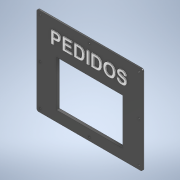
# Autodesk Inventor part: Front_Plate
Saved by Autodesk Inventor 2020 (Build 240168000, 168)
## iProperties
Created: 2020-06-21
Part Number: Front_Plate
Material: Generic
Document SubType Name: Modeling
Designer: Erick Miranda
Density: 1 g/cm^3
Appearance: Anodized - Black
Author: Erick Miranda
Autodesk Inventor part; units mm, degrees
ref_plane "YZ Plane" through (0, 0, 0) normal (1, 0, 0) x (0, 1, 0)
ref_plane "XZ Plane" through (0, 0, 0) normal (0, 1, 0) x (-1, 0, 0)
ref_plane "XY Plane" through (0, 0, 0) normal (0, 0, 1) x (1, 0, 0)
sketch "Sketch1" plane through (0, 0, 0) normal (0, 0, 1) x (1, 0, 0)
  line L0 (0, 0) -> (300, 0)
  line L1 (300, 0) -> (300, 250)
  line L2 (300, 250) -> (0, 250)
  line L3 (0, 250) -> (0, 0)
  dimension "d0" = 300
  dimension "d1" = 250
  constraints: 8 end point, 2 parallel, 1 horizontal, 1 perpendicular
  measures "d0" distance of L0.start L0.end
  measures "d1" distance of L0.end L1.end
extrude "Extrusion1" add sketch "Sketch1" along normal blind 4
fillet "Fillet1" radius 5 4 edges at (300, 250, 2) (0, 250, 2) (300, 0, 2) (0, 0, 2)
sketch "Sketch5" plane through (0, 0, 4) normal (0, 0, 1) x (1, 0, 0)
  line L0 (5, 0) -> (295, 0) projected
  line L1 (150, 0) -> (150, 33.5)
  line L2 (150, 33.5) -> (240.075, 33.5)
  line L3 (150, 33.5) -> (59.925, 33.5)
  line L4 (240.075, 33.5) -> (240.075, 155.5)
  line L5 (240.075, 155.5) -> (59.925, 155.5)
  line L6 (59.925, 155.5) -> (59.925, 33.5)
  point P0 (0, 0)
  dimension "d54" = 33.5
  dimension "d55" = 90.075
  dimension "d56" = 90.075
  dimension "d57" = 122
  dimension "d58" = 180.15
  constraints: 12 end point, 2 horizontal, 2 vertical, 1 midpoint, 1 perpendicular
  measures "d54" distance of L1.start L1.end
  measures "d55" distance of L1.end L2.end
  measures "d56" distance of L1.end L3.end
  measures "d57" distance of L2.end L4.end
  measures "d58" distance of L4.end L5.end
extrude "Extrusion5" cut sketch "Sketch5" against normal blind 81.3
chamfer "Chamfer2" distance 4 angle 45 4 edges at (240.075, 94.5, 4) (150, 33.5, 4) (150, 155.5, 4) (59.925, 94.5, 4)
sketch "Sketch7" plane through (0, 0, 4) normal (0, 0, 1) x (1, 0, 0)
  line L0 (38.9812, 222.1743) -> (264.0529, 222.1743) construction
  line L1 (264.0529, 222.1743) -> (264.0529, 185.0338) construction
  line L2 (264.0529, 185.0338) -> (38.9812, 185.0338) construction
  line L3 (38.9812, 185.0338) -> (38.9812, 222.1743) construction
  line L4 (42.5559, 186.5874) -> (42.5559, 221.5874)
  line L5 (42.5559, 221.5874) -> (53.8935, 221.5874)
  spline S0 degree 2 poles (53.8935, 221.5874) (60.3493, 221.5874) (62.2967, 221.0539) knots 0 0 0 1 1 1
  spline S1 degree 2 poles (62.2967, 221.0539) (65.3112, 220.2803) (69.3661, 214.9982) (69.3661, 210.81) knots 0 0 0 1 2 2 2
  spline S2 degree 2 poles (69.3661, 210.81) (69.3661, 207.6088) (67.0185, 203.2071) (63.4172, 200.6995) (61.5498, 200.2993) knots 0 0 0 1 2 3 3 3
  spline S3 degree 2 poles (61.5498, 200.2993) (59.0422, 199.7924) (54.2403, 199.7924) knots 0 0 0 1 1 1
  line L6 (54.2403, 199.7924) -> (49.6253, 199.7924)
  line L7 (49.6253, 199.7924) -> (49.6253, 186.5874)
  line L8 (49.6253, 186.5874) -> (42.5559, 186.5874)
  line L9 (49.6253, 215.6652) -> (49.6253, 205.7147)
  line L10 (49.6253, 205.7147) -> (53.4934, 205.7147)
  spline S4 degree 2 poles (53.4934, 205.7147) (57.6817, 205.7147) (60.4827, 206.8085) (62.0833, 209.156) (62.0833, 210.7033) knots 0 0 0 1 2 3 3 3
  spline S5 degree 2 poles (62.0833, 210.7033) (62.0833, 212.624) (59.8425, 215.1049) (58.1085, 215.4251) knots 0 0 0 1 2 2 2
  spline S6 degree 2 poles (58.1085, 215.4251) (56.8547, 215.6652) (53.0399, 215.6652) knots 0 0 0 1 1 1
  line L11 (53.0399, 215.6652) -> (49.6253, 215.6652)
  line L12 (75.1817, 186.5874) -> (75.1817, 221.5874)
  line L13 (75.1817, 221.5874) -> (101.1382, 221.5874)
  line L14 (101.1382, 221.5874) -> (101.1382, 215.6652)
  line L15 (101.1382, 215.6652) -> (82.251, 215.6652)
  line L16 (82.251, 215.6652) -> (82.251, 207.9022)
  line L17 (82.251, 207.9022) -> (99.831, 207.9022)
  line L18 (99.831, 207.9022) -> (99.831, 201.9799)
  line L19 (99.831, 201.9799) -> (82.251, 201.9799)
  line L20 (82.251, 201.9799) -> (82.251, 192.5097)
  line L21 (82.251, 192.5097) -> (101.8051, 192.5097)
  line L22 (101.8051, 192.5097) -> (101.8051, 186.5874)
  line L23 (101.8051, 186.5874) -> (75.1817, 186.5874)
  line L24 (107.7541, 221.5874) -> (120.6923, 221.5874)
  spline S7 degree 2 poles (120.6923, 221.5874) (125.0673, 221.5874) (127.3615, 220.9205) knots 0 0 0 1 1 1
  spline S8 degree 2 poles (127.3615, 220.9205) (130.4294, 220.0135) (134.831, 215.3717) (137.1253, 208.6758) (137.1253, 203.7406) knots 0 0 0 1 2 3 3 3
  spline S9 degree 2 poles (137.1253, 203.7406) (137.1253, 199.419) (136.0582, 196.2978) knots 0 0 0 1 1 1
  spline S10 degree 2 poles (136.0582, 196.2978) (134.7243, 192.483) (132.2967, 190.1088) knots 0 0 0 1 1 1
  spline S11 degree 2 poles (132.2967, 190.1088) (130.456, 188.3214) (127.3349, 187.3344) knots 0 0 0 1 1 1
  spline S12 degree 2 poles (127.3349, 187.3344) (124.9873, 186.5874) (121.0658, 186.5874) knots 0 0 0 1 1 1
  line L25 (121.0658, 186.5874) -> (107.7541, 186.5874)
  line L26 (107.7541, 186.5874) -> (107.7541, 221.5874)
  line L27 (114.8234, 215.6652) -> (114.8234, 192.5097)
  line L28 (114.8234, 192.5097) -> (120.1054, 192.5097)
  spline S13 degree 2 poles (120.1054, 192.5097) (123.0932, 192.5097) (124.4004, 192.8565) knots 0 0 0 1 1 1
  spline S14 degree 2 poles (124.4004, 192.8565) (126.1344, 193.2833) (128.4019, 195.3107) (129.8425, 200.0325) (129.8425, 204.0874) knots 0 0 0 1 2 3 3 3
  spline S15 degree 2 poles (129.8425, 204.0874) (129.8425, 208.1423) (128.4019, 212.4639) (125.8143, 214.8915) (123.8402, 215.3184) knots 0 0 0 1 2 3 3 3
  spline S16 degree 2 poles (123.8402, 215.3184) (122.3463, 215.6652) (117.998, 215.6652) knots 0 0 0 1 1 1
  line L29 (117.998, 215.6652) -> (114.8234, 215.6652)
  line L30 (142.8875, 186.5874) -> (142.8875, 221.5874)
  line L31 (142.8875, 221.5874) -> (149.9568, 221.5874)
  line L32 (149.9568, 221.5874) -> (149.9568, 186.5874)
  line L33 (149.9568, 186.5874) -> (142.8875, 186.5874)
  line L34 (156.6527, 221.5874) -> (169.591, 221.5874)
  spline S17 degree 2 poles (169.591, 221.5874) (173.966, 221.5874) (176.2602, 220.9205) knots 0 0 0 1 1 1
  spline S18 degree 2 poles (176.2602, 220.9205) (179.328, 220.0135) (183.7297, 215.3717) (186.0239, 208.6758) (186.0239, 203.7406) knots 0 0 0 1 2 3 3 3
  spline S19 degree 2 poles (186.0239, 203.7406) (186.0239, 199.419) (184.9568, 196.2978) knots 0 0 0 1 1 1
  spline S20 degree 2 poles (184.9568, 196.2978) (183.623, 192.483) (181.1954, 190.1088) knots 0 0 0 1 1 1
  spline S21 degree 2 poles (181.1954, 190.1088) (179.3547, 188.3214) (176.2335, 187.3344) knots 0 0 0 1 1 1
  spline S22 degree 2 poles (176.2335, 187.3344) (173.8859, 186.5874) (169.9644, 186.5874) knots 0 0 0 1 1 1
  line L35 (169.9644, 186.5874) -> (156.6527, 186.5874)
  line L36 (156.6527, 186.5874) -> (156.6527, 221.5874)
  line L37 (163.7221, 215.6652) -> (163.7221, 192.5097)
  line L38 (163.7221, 192.5097) -> (169.0041, 192.5097)
  spline S23 degree 2 poles (169.0041, 192.5097) (171.9919, 192.5097) (173.299, 192.8565) knots 0 0 0 1 1 1
  spline S24 degree 2 poles (173.299, 192.8565) (175.033, 193.2833) (177.3006, 195.3107) (178.7411, 200.0325) (178.7411, 204.0874) knots 0 0 0 1 2 3 3 3
  spline S25 degree 2 poles (178.7411, 204.0874) (178.7411, 208.1423) (177.3006, 212.4639) (174.7129, 214.8915) (172.7388, 215.3184) knots 0 0 0 1 2 3 3 3
  spline S26 degree 2 poles (172.7388, 215.3184) (171.2449, 215.6652) (166.8966, 215.6652) knots 0 0 0 1 1 1
  line L39 (166.8966, 215.6652) -> (163.7221, 215.6652)
  spline S27 degree 2 poles (190.5856, 203.874) (190.5856, 209.2094) (192.1862, 212.8374) knots 0 0 0 1 1 1
  spline S28 degree 2 poles (192.1862, 212.8374) (193.3867, 215.5051) (197.5216, 219.7734) (199.9759, 220.7871) knots 0 0 0 1 2 2 2
  spline S29 degree 2 poles (199.9759, 220.7871) (203.2304, 222.1743) (207.5254, 222.1743) knots 0 0 0 1 1 1
  spline S30 degree 2 poles (207.5254, 222.1743) (215.2617, 222.1743) (224.5452, 212.5707) (224.5452, 204.0341) knots 0 0 0 1 2 2 2
  spline S31 degree 2 poles (224.5452, 204.0341) (224.5452, 195.5775) (215.315, 186.0005) (207.6054, 186.0005) knots 0 0 0 1 2 2 2
  spline S32 degree 2 poles (207.6054, 186.0005) (199.8158, 186.0005) (190.5856, 195.5242) (190.5856, 203.874) knots 0 0 0 1 2 2 2
  spline S33 degree 2 poles (197.8684, 204.1141) (197.8684, 198.1652) (203.3638, 192.0295) (207.6054, 192.0295) knots 0 0 0 1 2 2 2
  spline S34 degree 2 poles (207.6054, 192.0295) (211.8471, 192.0295) (217.2625, 198.1118) (217.2625, 204.1941) knots 0 0 0 1 2 2 2
  spline S35 degree 2 poles (217.2625, 204.1941) (217.2625, 210.2231) (211.9804, 216.1453) (207.6054, 216.1453) knots 0 0 0 1 2 2 2
  spline S36 degree 2 poles (207.6054, 216.1453) (203.2304, 216.1453) (197.8684, 210.1431) (197.8684, 204.1141) knots 0 0 0 1 2 2 2
  line L40 (228.2533, 198.0051) -> (235.1359, 198.672)
  spline S37 degree 2 poles (235.1359, 198.672) (235.7495, 195.204) (239.5643, 191.9495) (242.7655, 191.9495) knots 0 0 0 1 2 2 2
  spline S38 degree 2 poles (242.7655, 191.9495) (246.1801, 191.9495) (249.6481, 194.8306) (249.6481, 196.778) knots 0 0 0 1 2 2 2
  spline S39 degree 2 poles (249.6481, 196.778) (249.6481, 198.0318) (248.1809, 199.7658) (246.3669, 200.406) knots 0 0 0 1 2 2 2
  spline S40 degree 2 poles (246.3669, 200.406) (245.1397, 200.8328) (240.7114, 201.9266) knots 0 0 0 1 1 1
  spline S41 degree 2 poles (240.7114, 201.9266) (235.0292, 203.3405) (232.735, 205.3946) knots 0 0 0 1 1 1
  spline S42 degree 2 poles (232.735, 205.3946) (229.5071, 208.2757) (229.5071, 212.4106) knots 0 0 0 1 1 1
  spline S43 degree 2 poles (229.5071, 212.4106) (229.5071, 215.1049) (232.5483, 219.7467) (238.2571, 222.1743) (242.2853, 222.1743) knots 0 0 0 1 2 3 3 3
  spline S44 degree 2 poles (242.2853, 222.1743) (248.8745, 222.1743) (255.5437, 216.4121) (255.7038, 211.5836) knots 0 0 0 1 2 2 2
  line L41 (255.7038, 211.5836) -> (248.6344, 211.2635)
  spline S45 degree 2 poles (248.6344, 211.2635) (248.1809, 213.9578) (245.1931, 216.3321) (242.2053, 216.3321) knots 0 0 0 1 2 2 2
  spline S46 degree 2 poles (242.2053, 216.3321) (239.1108, 216.3321) (237.3768, 215.0783) knots 0 0 0 1 1 1
  spline S47 degree 2 poles (237.3768, 215.0783) (236.2564, 214.2513) (236.2564, 212.8908) knots 0 0 0 1 1 1
  spline S48 degree 2 poles (236.2564, 212.8908) (236.2564, 211.6636) (237.2967, 210.7566) knots 0 0 0 1 1 1
  spline S49 degree 2 poles (237.2967, 210.7566) (238.6573, 209.6362) (248.9812, 207.2086) (253.9164, 204.621) (256.7175, 200.1126) (256.7175, 196.778) knots 0 0 0 1 2 3 4 4 4
  spline S50 degree 2 poles (256.7175, 196.778) (256.7175, 193.7902) (253.3829, 188.5348) (247.2739, 185.9739) (242.7121, 185.9739) knots 0 0 0 1 2 3 3 3
  spline S51 degree 2 poles (242.7121, 185.9739) (236.0696, 185.9739) (228.9469, 192.1095) (228.2533, 198.0051) knots 0 0 0 1 2 2 2
  point P0 (0, 0)
  constraints: 2 other
sketch "Sketch8" plane through (0, 0, 4) normal (0, 0, 1) x (1, 0, 0)
  line L0 (5, 250) -> (0, 250)
  arc A0 (5, 250) -> (0, 245) centre (5, 245) ccw projected
  line L1 (0, 250) -> (0, 245)
  line L2 (0, 245) -> (0, 5) projected
  line L3 (0, 245) -> (0, 240)
  line L4 (0, 240) -> (10, 240)
  circle A1 centre (10, 240) radius 2.5
  line L5 (295, 250) -> (5, 250) projected
  line L6 (150, 250) -> (150, 0)
  line L7 (5, 0) -> (295, 0) projected
  line L8 (295, 250) -> (300, 250)
  arc A2 (300, 245) -> (295, 250) centre (295, 245) ccw
  line L9 (300, 250) -> (300, 245)
  line L10 (300, 245) -> (300, 240)
  line L11 (300, 240) -> (290, 240)
  circle A3 centre (290, 240) radius 2.5
  line L12 (0, 125) -> (300, 125)
  line L13 (300, 5) -> (300, 245) projected
  line L14 (5, 0) -> (0, 0)
  arc A4 (0, 5) -> (5, 0) centre (5, 5) ccw
  line L15 (0, 0) -> (0, 5)
  line L16 (0, 5) -> (0, 10)
  line L17 (0, 10) -> (10, 10)
  circle A5 centre (10, 10) radius 2.5
  line L18 (295, 0) -> (300, 0)
  arc A6 (295, 0) -> (300, 5) centre (295, 5) ccw
  line L19 (300, 0) -> (300, 5)
  line L20 (300, 5) -> (300, 10)
  line L21 (300, 10) -> (290, 10)
  circle A7 centre (290, 10) radius 2.5
  line L22 (150, 250) -> (150, 240)
  circle A8 centre (150, 240) radius 2.5
  line L23 (150, 0) -> (150, 10)
  circle A9 centre (150, 10) radius 2.5
  line L24 (300, 125) -> (290, 125)
  circle A10 centre (290, 125) radius 2.5
  line L25 (0, 125) -> (10, 125)
  circle A11 centre (10, 125) radius 2.5
  point P0 (0, 0)
  dimension "d70" = 5
  dimension "d71" = 10
  dimension "d72" = 5
  dimension "d81" = 10
  dimension "d82" = 5
  dimension "d83" = 10
  dimension "d84" = 5
  dimension "d85" = 10
  dimension "d86" = 5
  dimension "d87" = 10
  dimension "d88" = 5
  constraints: 44 end point, 16 symmetric about line, 11 centre point, 8 coincident, 6 point on circle, 5 point on line, 4 midpoint, 2 perpendicular, 1 horizontal, 1 tangent, 6 other
  measures "d70" distance of L1.end L3.end
  measures "d71" distance of L3.end L4.end
  measures "d72" diameter of A1
  measures "d81" distance of L6.start L22.end
  measures "d82" diameter of A8
  measures "d83" distance of L6.end L23.end
  measures "d84" diameter of A9
  measures "d85" distance of L12.end L24.end
  measures "d86" diameter of A10
  measures "d87" distance of L12.start L25.end
  measures "d88" diameter of A11
extrude "Extrusion6" cut sketch "Sketch8" against normal blind 81.3 contours A1 | A3 | A8 L6 | L6 A8 | A5 | A11 L12 | L12 A11 | A7 | A9 L6 | L6 A9 | A10 L12 | L12 A10
extrude "Extrusion7" add sketch "Sketch7" along normal blind 2
sketch "Front-CNC-CUT" plane through (0, 0, 4) normal (0, 0, 1) x (1, 0, 0)
  circle A0 centre (10, 240) radius 2.6
  circle A1 centre (290, 240) radius 2.6
  circle A2 centre (290, 10) radius 2.6
  circle A3 centre (10, 10) radius 2.6
  arc A4 (0, 5) -> (5, 0) centre (5, 5) ccw projected
  arc A5 (0, 5) -> (5, 0) centre (5, 5) ccw
  arc A6 (5, 250) -> (0, 245) centre (5, 245) ccw projected
  arc A7 (5, 250) -> (0, 245) centre (5, 245) ccw
  arc A8 (300, 245) -> (295, 250) centre (295, 245) ccw projected
  arc A9 (300, 245) -> (295, 250) centre (295, 245) ccw
  arc A10 (295, 0) -> (300, 5) centre (295, 5) ccw projected
  arc A11 (295, 0) -> (300, 5) centre (295, 5) ccw
  line L0 (300, 5) -> (300, 245) projected
  line L1 (300, 5) -> (300, 245)
  line L2 (295, 250) -> (5, 250) projected
  line L3 (295, 250) -> (5, 250)
  line L4 (0, 245) -> (0, 5)
  line L5 (5, 0) -> (295, 0) projected
  line L6 (5, 0) -> (295, 0)
  circle A12 centre (150, 240) radius 2.6
  circle A13 centre (150, 10) radius 2.6
  circle A14 centre (290, 125) radius 2.6
  circle A15 centre (10, 125) radius 2.5 projected
  circle A16 centre (10, 125) radius 2.6
  point P0 (0, 0)
  dimension "d93" = 250
  dimension "d94" = 300
  constraints: 12 centre point, 8 coincident, 8 end point, 8 point on circle, 6 tangent, 3 collinear, 1 concentric, 1 vertical
  measures "d93" distance between parallel lines of L5 L2
  measures "d94" distance between parallel lines of L0 L4
body "Solid1"
